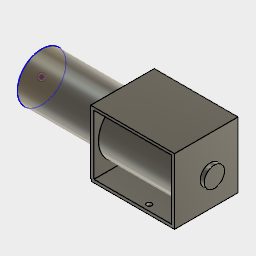
Winch v4 (Autodesk Fusion 360 design; units mm, degrees)
Autodesk Fusion 360 part; units mm, degrees
sketch "Sketch1" plane through (0, 0, 0) normal (1, 0, 0) x (0, 1, 0)
  circle A0 centre (0, 0) radius 38.1
  dimension "d1" = 76.2
  measures "d1" diameter of A0
extrude "Extrude2" add sketch "Sketch1" along normal blind 127 makes body 1
sketch "Sketch3" plane through (127, 0, 0) normal (1, 0, 0) x (0, 1, 0)
  circle A0 centre (0, 0) radius 38.1
  line L0 (-50.0062, 50.0063) -> (50.0063, 50.0063)
  line L1 (50.0063, 50.0063) -> (50.0062, -50.0063)
  line L2 (50.0062, -50.0063) -> (-50.0062, -50.0063)
  line L3 (-50.0062, -50.0063) -> (-50.0062, 50.0063)
  line L4 (-50.0062, 50.0063) -> (50.0062, -50.0063) construction
  dimension "d17" = 100.0125
  constraint horizontal L0
  constraint vertical L1
  constraint horizontal L2
  constraint vertical L3
  constraint midpoint L4
  constraint equal L0 L3
extrude "Extrude3" add sketch "Sketch3" along normal blind 131.7625 contours A0 | L0 L1 L2 L3 bodies 1
sketch "Sketch4" plane through (258.7625, 0, 0) normal (1, 0, 0) x (0, 1, 0)
  line L0 (-50.0062, -50.0063) -> (50.0062, -50.0063)
  line L1 (50.0062, -50.0063) -> (50.0063, 50.0063)
  line L2 (50.0063, 50.0063) -> (-50.0062, 50.0063)
  line L3 (-50.0062, 50.0063) -> (-50.0062, -50.0063)
  circle A0 centre (0, 0) radius 1.8161
extrude "Extrude4" add sketch "Sketch4" along normal blind 6.35 contours A0 bodies 1
sketch "Sketch5" plane through (265.1125, 0, 0) normal (1, 0, 0) x (0, 1, 0)
  circle A0 centre (0, 0) radius 1.8161
  circle A1 centre (0, 0) radius 15.875
  dimension "d10" = 31.75
  measures "d10" diameter of A1
extrude "Extrude5" add sketch "Sketch5" along normal blind 6.35 separate body contours A0 | A1 makes body 2
sketch "Sketch6" plane through (0, 0, -50.0063) normal (0, 0, -1) x (1, 0, 0)
  line L0 (127, 50.0062) -> (127, -50.0062)
  line L1 (127, -50.0062) -> (258.7625, -50.0062)
  line L2 (258.7625, -50.0062) -> (258.7625, 50.0062)
  line L3 (258.7625, 50.0062) -> (127, 50.0062)
  line L4 (128.5875, 50.0062) -> (258.7625, 50.0062)
  line L5 (258.7625, 50.0062) -> (258.7625, -50.0063)
  line L6 (258.7625, -50.0063) -> (128.5875, -50.0063)
  line L7 (128.5875, -50.0063) -> (128.5875, 50.0062)
  circle A0 centre (209.55, 40.4812) radius 3.9688
  circle A1 centre (209.55, -40.4813) radius 3.9688
  dimension "d13" = 130.175
  dimension "d14" = 100.0125
  dimension "d18" = 7.9375
  dimension "d19" = 80.9625
  dimension "d20" = 9.525
  dimension "d21" = 80.9625
  constraint horizontal L4
  constraint vertical L5
  constraint horizontal L6
  constraint vertical L7
  constraint equal A0 A1
  measures "d18" diameter of A0
  measures "d19" distance of L7
  measures "d20" distance of L4
extrude "Extrude6" add sketch "Sketch6" along normal blind 3.175 contours L1 L2 L3 L4 L5 L6 L7 bodies 1
sketch "Sketch7" plane through (0, -50.0062, 0) normal (0, -1, 0) x (1, 0, 0)
  line L0 (127, 50.0063) -> (127, -50.0063)
  line L1 (127, -50.0063) -> (128.5875, -50.0063)
  line L2 (128.5875, -50.0063) -> (128.5875, -53.1812)
  line L3 (128.5875, -53.1813) -> (258.7625, -53.1813)
  line L4 (258.7625, -53.1813) -> (258.7625, 50.0063)
  line L5 (258.7625, 50.0063) -> (127, 50.0063)
  line L6 (254, 45.72) -> (132.08, 45.72)
  line L7 (132.08, 45.72) -> (132.08, -48.26)
  line L8 (132.08, -48.26) -> (254, -48.26)
  line L9 (254, -48.26) -> (254, 45.72)
  constraint horizontal L6
  constraint vertical L7
  constraint horizontal L8
  constraint vertical L9
extrude "Extrude7" cut sketch "Sketch7" against normal up to surface (100.0125 mm away) contours L6 L7 L8 L9 bodies 1
extrude "Extrude8" cut 2 faces at (208.8746, -40.0913, -50.0063) (208.3446, 40.4813, -50.0063) along direction (0, 0, -1) up to surface end surface through (132.08, -50.0062, -48.26) normal (0, 0, 1) offset 0 on bodies 1 bodies 1
sketch "Sketch8" plane through (132.08, 0, 0) normal (1, 0, 0) x (0, 1, 0)
  line L0 (50.0062, -48.26) -> (50.0063, 45.72)
  line L1 (50.0063, 45.72) -> (-50.0062, 45.72)
  line L2 (-50.0062, 45.72) -> (-50.0062, -48.26)
  line L3 (-50.0062, -48.26) -> (50.0062, -48.26)
  circle A0 centre (0, 0) radius 42.7015
extrude "Extrude9" add sketch "Sketch8" along normal up to surface (121.92 mm away) contours A0 bodies 1
equation "d6 = 5 in + ( 3 / 16 ) * 1 in"
equation "d14 = 3 in + ( 15 / 16 ) * 1 in"
equation "d15 = ( 1 / 8 ) * 1 in"
equation "d17 = 3 in + ( 15 / 16 ) * 1 in"
equation "d18 = ( 5 / 16 ) * 1 in"
equation "d19 = 3 in + ( 3 / 16 ) * 1 in"
equation "d20 = ( 3 / 8 ) * 1 in"
equation "d21 = 3 in + ( 3 / 16 ) * 1 in"
